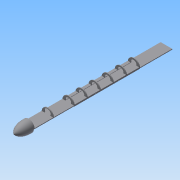
# Autodesk Inventor part: konstruksi roket
Saved by Autodesk Inventor 2014 SP1 (Build 180222100, 222)
## iProperties
Created: 2018-05-28
Part Number: konstruksi roket
Material: Generic
Document SubType Name: Modeling
Designer: Dadang
Density: 1 g/cm^3
Appearance: Default
Author: Dadang
Autodesk Inventor part; units mm, degrees
ref_plane "XY Plane" through (0, 0, 0) normal (0, 0, 1) x (1, 0, 0)
sketch "Sketch1" plane through (0, 0, 0) normal (0, 0, 1) x (1, 0, 0)
  line L0 (955, 0) -> (955, 80)
  line L1 (0, 80) -> (0, 0)
  line L2 (277, 0) -> (277, 20)
  line L3 (277, 20) -> (733, 20)
  line L4 (733, 20) -> (733, 0)
  line L5 (277, 80) -> (277, 60)
  line L6 (277, 60) -> (733, 60)
  line L7 (733, 60) -> (733, 80)
  line L8 (0, 80) -> (955, 80)
  line L9 (427, 0) -> (427, 20)
  line L10 (583, 0) -> (583, 20)
  line L11 (0, 0) -> (955, 0)
  line L12 (277, 0) -> (733, 0)
  line L13 (733, 80) -> (277, 80)
  dimension "d0" = 955
  dimension "d1" = 80
  dimension "d2" = 277
  dimension "d3" = 20
  dimension "d4" = 456
  dimension "d5" = 150
  dimension "d6" = 150
  constraints: 28 end point, 3 perpendicular, 2 collinear, 2 parallel, 2 point on line
  measures "d0" distance of L1.start L0.end
  measures "d1" distance of L0.end L0.start
  measures "d2" distance of L1.end L2.start
  measures "d3" distance of L2.start L2.end
  measures "d4" distance of L2.end L3.end
  measures "d5" distance of L2.start L9.start
  measures "d6" distance of L4.end L10.start
extrude "Extrusion1" add sketch "Sketch1" along normal mid plane 5 contours L11 L4 L3 L2 L1 L8 L5 L6 L7 L0
extrude "Extrusion2" add sketch "Sketch1" along normal mid plane 10 contours L11 L10 L3 L4 | L7 L6 L5 L8 | L11 L9 L3 L10 | L11 L2 L3 L9
sketch "Sketch3" plane through (0, 0, 2.5) normal (-1, 0, 0) x (0, 0, 1)
  line L0 (-5, 0) -> (-5, 80) projected
  arc A0 (0, 0.0782) -> (0, 79.9218) centre (-2.5, 40) ccw
  arc A1 (0, 20.0782) -> (0, 59.9218) centre (10.4691, 40) ccw
  line L1 (0, 79.9218) -> (0, 59.9218)
  line L2 (0, 20.0782) -> (0, 0.0782)
  point P0 (-2.5, 0)
  dimension "d18" = 20
  dimension "d19" = 20
  constraints: 4 end point, 4 point on circle, 2 centre point, 1 collinear, 1 parallel
  measures "d18" distance of L1.start L1.end
  measures "d19" distance of L2.end L2.start
extrude "Extrusion4" add sketch "Sketch3" against normal blind 5
pattern_linear "Rectangular Pattern1" count 2 spacing 133.5 along (1, 0, 0) of "Extrusion4"
ref_plane "Work Plane1" through (277, 0, 0) normal (1, 0, 0) x (0, 1, 0)
sketch "Sketch4" plane through (277, 0, 0) normal (1, 0, 0) x (0, 1, 0)
  line L0 (80, 2.5) -> (80, -2.5) projected
  line L1 (80, -5) -> (80, -2.5) projected
  line L2 (80, -2.5) -> (80, -5) projected
  line L3 (80, 2.5) -> (80, -2.5) projected
  line L4 (80, 5) -> (80, 2.5) projected
  line L5 (80, 2.5) -> (80, 5) projected
  line L6 (0, 2.5) -> (0, -2.5) projected
  line L7 (0, 5) -> (0, 2.5) projected
  line L8 (0, 2.5) -> (0, 5) projected
  line L9 (0, -2.5) -> (0, 2.5) projected
  line L10 (0, -5) -> (0, -2.5) projected
  line L11 (0, -2.5) -> (0, -5) projected
  line L12 (80, 5) -> (60, 5) projected
  line L13 (60, 5) -> (80, 5) projected
  line L14 (20, 5) -> (0, 5) projected
  line L15 (0, 5) -> (20, 5) projected
  line L16 (60, 2.5) -> (60, 5) projected
  line L17 (60, 2.5) -> (60, 5) projected
  line L18 (20, 5) -> (20, 2.5) projected
  line L19 (20, 5) -> (20, 2.5) projected
  line L20 (78.7298, 5) -> (60, 5)
  line L21 (20, 5) -> (0.9311, 5)
  line L22 (20, 5) -> (20, 2.5)
  line L23 (60, 5) -> (60, 2.5)
  arc A0 (60, 5) -> (20, 5) centre (40, 9.7482) ccw
  line L24 (20, -2.5) -> (20, -5) projected
  line L25 (20, -2.5) -> (20, -5) projected
  line L26 (60, -5) -> (60, -2.5) projected
  line L27 (60, -5) -> (60, -2.5) projected
  arc A1 (80, 0) -> (0, 0) centre (40, 0) ccw
  line L28 (79.6863, 5) -> (60, 5)
  line L29 (20, 5) -> (0.3137, 5)
  line L30 (0.3137, 5) -> (0, 5)
  line L31 (0, 5) -> (0, 0)
  line L32 (79.6863, 5) -> (80, 5)
  line L33 (80, 5) -> (80, 0)
  point P0 (80, 5)
  point P1 (80, -5)
  point P2 (0, -5)
  point P3 (0, 5)
  dimension "d26" = 80
  constraints: 20 end point, 7 collinear, 6 point on circle, 4 point on line, 2 centre point, 1 midpoint, 1 tangent
  measures "d26" diameter of A1
extrude "Extrusion5" add sketch "Sketch4" along normal blind 5 contours L12 A0 L14 A1
extrude "Extrusion6" cut sketch "Sketch4" along normal blind 500 contours A1 L6 L7 L14 | L0 A1 L12 L4
sketch "Sketch5" plane through (277, 0, -5) normal (0, -1, 0) x (1, 0, 0)
  circle A0 centre (306, 5) radius 2.5
  circle A1 centre (150, 5) radius 2.5
  point P0 (-277, 5)
  dimension "d33" = 5
  dimension "d34" = 5
  constraints: 2 centre point
  measures "d33" diameter of A0
  measures "d34" diameter of A1
extrude "Extrusion7" cut sketch "Sketch5" against normal blind 500
pattern_linear "Rectangular Pattern2" count 6 spacing 90.2 along (1, 0, 0) of "Extrusion5"
ref_plane "Work Plane2" through (0, 40, 0) normal (0, 1, 0) x (-1, 0, 0)
sketch "Sketch6" plane through (0, 40, 0) normal (0, 1, 0) x (-1, 0, 0)
  line L0 (0, -2.5) -> (0, 2.5) projected
  line L1 (0, 2.5) -> (0, 40) projected
  line L2 (0, 0) -> (100, 0)
  spline S0 degree 4 poles (0, 40) (18.8191, 40.6892) (34.5273, 38.677) (78.4206, 36.7816) (100, 0) knots 0 0 0 0 0 1 1 1 1 1
  line L3 (0, 40) -> (0, 0)
  point P0 (13.5096, 40)
  point P1 (31.8449, 38.4324)
  point P2 (61.8997, 30.8714)
  dimension "d41" = 100
  constraints: 4 end point, 1 collinear, 1 perpendicular, 5 other
  measures "d41" distance of L2.start L2.end
revolve "Revolution1" add sketch "Sketch6" angle 360 about axis through (0, 40, 0) along (-1, 0, 0)
body "Solid1"
